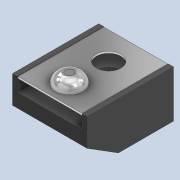
# Autodesk Inventor part: High Voltage Limit Switch Arm Coupler
Saved by Autodesk Inventor 2022 (Build 260153000, 153)
## iProperties
Created: 2021-10-24
Part Number: High Voltage Limit Switch Arm Coupler
Material: Generic
Document SubType Name: Modeling
Designer: Coy
Density: 1 g/cm^3
Appearance: Chrome - Polished
Author: Coy
Autodesk Inventor part; units mm, degrees
ref_plane "YZ Plane" through (0, 0, 0) normal (1, 0, 0) x (0, 1, 0)
ref_plane "XZ Plane" through (0, 0, 0) normal (0, 1, 0) x (-1, 0, 0)
ref_plane "XY Plane" through (0, 0, 0) normal (0, 0, 1) x (1, 0, 0)
sketch "Sketch1" plane through (0, 0, 0) normal (0, 0, 1) x (1, 0, 0)
  line L0 (0, 0) -> (-19, 0)
  line L1 (-19, 0) -> (-19, 12)
  line L2 (-19, 12) -> (0, 12)
  line L3 (0, 12) -> (0, 0)
  line L4 (-17.75, 12) -> (-1.25, 12)
  line L5 (-1.25, 12) -> (-1.25, 8.5)
  line L6 (-1.25, 8.5) -> (-17.75, 8.5)
  line L7 (-17.75, 8.5) -> (-17.75, 12)
  point P0 (-1.25, 12)
  dimension "d0" = 19
  dimension "d1" = 12
  dimension "d2" = 16.5
  dimension "d3" = 3.5
  dimension "d4" = 1.25
  constraints: 16 end point, 4 parallel, 2 horizontal, 2 perpendicular, 1 point on line
  measures "d0" distance of L1.end L2.end
  measures "d1" distance of L0.end L1.end
  measures "d2" distance of L5.end L6.end
  measures "d3" distance of L4.end L5.end
  measures "d4" distance between parallel lines of L1 L7
extrude "Extrusion1" add sketch "Sketch1" against normal blind 22 contours L0 L1 L2 L7 L6 L5 L3
chamfer "Chamfer1" distance 5 distance2 8 1 edges at (-9.5, 0, 0) measured on face at (-6.75, 2.8333, 0)
sketch "Sketch2" plane through (-19, 0, -22) normal (0, -1, 0) x (1, 0, 0)
  line L0 (0, 14) -> (19, 14) construction
  line L1 (9.5, 14) -> (9.5, 0) construction
  line L2 (1.25, 0) -> (17.75, 0) construction
  circle A0 centre (9.5, 7) radius 3.125
  point P0 (19, 22)
  dimension "d10" = 6.25
  constraints: 3 midpoint, 2 end point, 1 centre point
  measures "d10" diameter of A0
extrude "Extrusion2" cut sketch "Sketch2" against normal up to next
sketch "Sketch3" plane through (-19, 12, 0) normal (0, 1, 0) x (1, 0, 0)
  circle A0 centre (9.5, 15) radius 3.125 projected
  line L0 (17.75, 0) -> (1.25, 0) projected
  line L1 (17.75, 0) -> (17.75, 22) projected
  line L2 (1.25, 22) -> (17.75, 22) projected
  line L3 (1.25, 0) -> (1.25, 22) projected
  line L4 (1.35, 21.9) -> (17.65, 21.9)
  line L5 (17.65, 21.9) -> (17.65, 0.1)
  line L6 (17.65, 0.1) -> (1.35, 0.1)
  line L7 (1.35, 0.1) -> (1.35, 21.9)
  point P0 (19, 0)
  dimension "d13" = 0.1
  constraints: 8 end point, 3 other
  measures "d13" distance between parallel lines of L3 L7
extrude "Extrusion3" add sketch "Sketch3" against normal blind 0.5 contours L4 L5 L6 L7
sketch "Sketch4" plane through (-19, 12, 0) normal (0, 1, 0) x (1, 0, 0)
  line L0 (17.65, 0.1) -> (1.35, 0.1) construction
  line L1 (9.5, 0.1) -> (9.5, 21.9) construction
  line L2 (17.65, 21.9) -> (1.35, 21.9) construction
  circle A0 centre (9.5, 5) radius 3.5
  circle A1 centre (9.5, 15) radius 3.125 projected
  point P0 (19, 0)
  dimension "d16" = 7
  dimension "d17" = 10
  constraints: 2 end point, 2 midpoint, 1 centre point, 1 point on line
  measures "d16" diameter of A0
  measures "d17" distance of A1.centre A0.centre
extrude "Extrusion4" add sketch "Sketch4" along normal blind 2.5 contours A0
fillet "Fillet1" radius 2.5 1 edges at (-13, 14.5, -5)
sketch "Sketch5" plane through (-19, 0, -22) normal (-1, 0, 0) x (0, 0, 1)
  line L0 (7, 12) -> (7, 0) construction
  line L1 (22, 5) -> (14, 0) construction
  line L2 (22, 12) -> (22, 5) construction
  line L3 (22, 12) -> (0, 12) construction
  line L4 (0, 0) -> (0, 12) construction
  line L5 (14, 0) -> (0, 0) construction
  circle A0 centre (7, 6) radius 2.875
  point P0 (22, 0)
  dimension "d21" = 5.75
  constraints: 2 end point, 2 midpoint, 1 centre point, 1 point on line, 1 vertical
  measures "d21" diameter of A0
extrude "Extrusion5" add sketch "Sketch5" along normal blind 1.5
equation "\"d4\" = -0.5 * d2 + 0.5 * d0"
body "Solid1"
